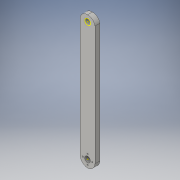
# Autodesk Inventor part: BB-8_headslider_rod
Saved by Autodesk Inventor 2016 (Build 200138000, 138)
## iProperties
Created: 2018-07-19
Part Number: BB-8_headslider_rod
Material: Generic
Document SubType Name: Modeling
Designer: Karcsi
Density: 1 g/cm^3
Appearance: Default
Author: Karcsi
Autodesk Inventor part; units mm, degrees
ref_plane "YZ Plane" through (0, 0, 0) normal (1, 0, 0) x (0, 1, 0)
ref_plane "XZ Plane" through (0, 0, 0) normal (0, 1, 0) x (-1, 0, 0)
ref_plane "XY Plane" through (0, 0, 0) normal (0, 0, 1) x (1, 0, 0)
sketch "Sketch1" plane through (0, 0, 0) normal (0, 0, 1) x (1, 0, 0)
  arc A0 (10.5, 0) -> (0, -10.5) centre (0, 0) ccw
  circle A1 centre (0, 8) radius 0.5
  circle A2 centre (-8, 0) radius 0.5
  circle A3 centre (0, -8) radius 0.5
  circle A4 centre (8, 0) radius 0.5
  line L0 (-10.5, 0) -> (-12.5, 0) construction
  arc A5 (0, -10.5) -> (10.5, 0) centre (0, 0) ccw
  line L1 (10.5, 0) -> (12.5, 0)
  line L2 (0, -10.5) -> (0, -12.5) construction
  arc A6 (-12.5, 0) -> (0, -12.5) centre (0.4907, 0.4907) ccw
  arc A7 (0, -12.5) -> (12.5, 0) centre (-0.4907, 0.4907) ccw
  line L3 (-12.5, 0) -> (12.5, 0) construction
  line L4 (12.5, 0) -> (12.5, 200)
  line L5 (12.5, 200) -> (-12.5, 200) construction
  line L6 (-12.5, 200) -> (-12.5, 0)
  arc A8 (4.85, 200) -> (-4.85, 200) centre (0, 200) ccw
  line L7 (0, 200) -> (0, 210) construction
  arc A9 (0, 210) -> (-12.5, 200) centre (-0.6647, 198.0184) ccw
  arc A10 (12.5, 200) -> (0, 210) centre (0.6647, 198.0184) ccw
  arc A11 (-4.85, 200) -> (4.85, 200) centre (0, 200) ccw
  dimension "d0" = 21
  dimension "d1" = 1
  dimension "d2" = 1
  dimension "d3" = 1
  dimension "d4" = 1
  dimension "d5" = 8
  dimension "d6" = 8
  dimension "d7" = 8
  dimension "d8" = 8
  dimension "d14" = 12.5
  dimension "d15" = 12.5
  dimension "d16" = 12.5
  dimension "d17" = 2
  dimension "d18" = 2
  dimension "d19" = 2
  dimension "d20" = 13
  dimension "d21" = 13
  dimension "d30" = 200
  dimension "d31" = 9.7
  dimension "d32" = 12.5
  dimension "d34" = 2.5
  dimension "d35" = 2.5
  dimension "d36" = 2.5
  dimension "d37" = 10
  dimension "d38" = 12
  dimension "d39" = 12
  constraints: 17 point on circle, 16 end point, 12 centre point, 3 horizontal, 2 parallel, 2 point on line, 2 vertical, 1 coincident, 1 midpoint, 1 perpendicular
  measures "d0" diameter of A0
  measures "d1" diameter of A1
  measures "d2" diameter of A2
  measures "d3" diameter of A3
  measures "d4" diameter of A4
  measures "d5" distance of point (0, 0) A1.centre
  measures "d6" distance of point (0, 0) A4.centre
  measures "d7" distance of point (0, 0) A3.centre
  measures "d8" distance of point (0, 0) A2.centre
  measures "d14" distance of A0.centre L0.end
  measures "d15" distance of A0.centre L1.end
  measures "d16" distance of A0.centre L2.end
  measures "d17" distance of L1.start L1.end
  measures "d18" distance of L0.start L0.end
  measures "d19" distance of L2.start L2.end
  measures "d20" radius of A6
  measures "d21" radius of A7
  measures "d30" distance of L4.end L3.end
  measures "d31" diameter of A8
  measures "d32" distance of L5.end L7.start
  measures "d34" distance of L2.start A3.centre
  measures "d35" distance of L0.start A2.centre
  measures "d36" distance of L1.start A4.centre
  measures "d37" distance of L7.start L7.end
  measures "d38" radius of A9
  measures "d39" radius of A10
sketch "Sketch2" plane through (0, 0, 0) normal (0, 0, 1) x (1, 0, 0)
  arc A0 (10.5, 0) -> (0, -10.5) centre (0, 0) ccw projected
  circle A1 centre (-8, 0) radius 0.5 projected
  circle A2 centre (0, -8) radius 0.5 projected
  circle A3 centre (8, 0) radius 0.5 projected
  circle A4 centre (0, 8) radius 0.5 projected
  arc A5 (0, -10.5) -> (10.5, 0) centre (0, 0) ccw projected
sketch "Sketch3" plane through (0, 0, 0) normal (0, 0, 1) x (1, 0, 0)
  arc A0 (0, 210) -> (-12.5, 200) centre (-0.6647, 198.0184) ccw projected
  line L0 (-12.5, 200) -> (-12.5, 0) projected
  arc A1 (-12.5, 0) -> (0, -12.5) centre (0.4907, 0.4907) ccw projected
  arc A2 (0, -12.5) -> (12.5, 0) centre (-0.4907, 0.4907) ccw projected
  line L1 (12.5, 0) -> (12.5, 200) projected
  arc A3 (12.5, 200) -> (0, 210) centre (0.6647, 198.0184) ccw projected
  point P0 (0, 0)
extrude "Extrusion1" add sketch "Sketch3" along normal blind 8.2
extrude "Extrusion2" cut sketch "Sketch1" along normal blind 10 contours A11 A8
extrude "Extrusion3" cut sketch "Sketch2" along normal blind 2
sketch "Sketch4" plane through (8, 0, 0) normal (0, 0, -1) x (-1, 0, 0)
  circle A0 centre (0, 0) radius 0.5 projected
  circle A1 centre (8, 8) radius 0.5 projected
  circle A2 centre (16, 0) radius 0.5 projected
  circle A3 centre (8, -8) radius 0.5 projected
  point P0 (8, 0)
hole "Hole1" at (0, 8, 0) at (8, 0, 0) at (0, -8, 0) at (-8, 0, 0) direction (0, 0, 1) diameter 2 depth 10 tip angle 118
sketch "Sketch5" plane through (0, 0, 8.2) normal (0, 0, 1) x (1, 0, 0)
  point P0 (0, 0)
sketch "Sketch6" plane through (0, 0, 8.2) normal (0, 0, 1) x (1, 0, 0)
  circle A0 centre (0, 200) radius 4.85 projected
  point P0 (0, 0)
sketch "Sketch7" plane through (0, 0, 8.2) normal (0, 0, 1) x (1, 0, 0)
  point P0 (0, 0)
sketch "Sketch9" plane through (0, 0, 0) normal (0, 0, -1) x (-1, 0, 0)
  circle A0 centre (0, 0) radius 10.75
  dimension "d55" = 21.5
  constraints: 1 centre point, 1 coincident
  measures "d55" diameter of A0
extrude "Extrusion5" cut sketch "Sketch9" against normal blind 2
sketch "Sketch10" plane through (0, 0, 2) normal (0, 0, -1) x (-1, 0, 0)
  circle A0 centre (0, 0) radius 4.75
  dimension "d58" = 9.5
  constraints: 1 centre point, 1 coincident
  measures "d58" diameter of A0
extrude "Extrusion6" cut sketch "Sketch10" against normal blind 10
body "Solid1"
